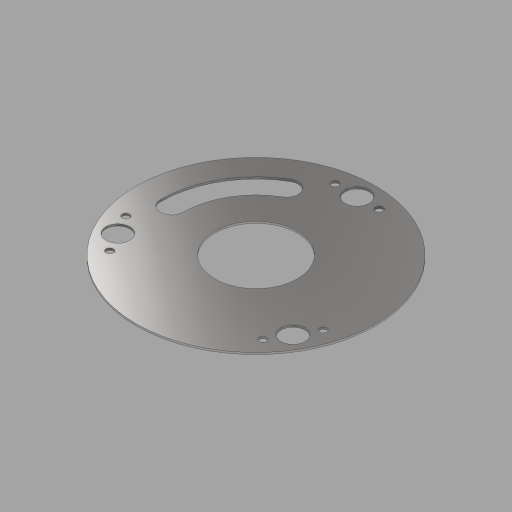
# Autodesk Inventor part: Baffle
Saved by Autodesk Inventor 2024 (Build 280153020, 153B)
## iProperties
Created: 2023-10-26
Part Number: Baffle
Material: Stainless Steel
Document SubType Name: Modeling
Designer: schanen
Density: 8 g/cm^3
Appearance: Semi-Polished
Mass: 11.1966 g
Surface Area: 231.347 cm^2
Volume: 11.1966 cm^3
baffle_or: 65.000 mm
tubes_r: 55.000 mm
Author: schanen
Autodesk Inventor part; units mm, degrees
ref_plane "YZ Plane" through (0, 0, 0) normal (1, 0, 0) x (0, 1, 0)
ref_plane "XZ Plane" through (0, 0, 0) normal (0, 1, 0) x (-1, 0, 0)
ref_plane "XY Plane" through (0, 0, 0) normal (0, 0, 1) x (1, 0, 0)
sketch "Sketch1" plane through (0, 0, 0) normal (0, 0, 1) x (1, 0, 0)
  line L0 (0, 0) -> (-65, 0)
  line L1 (-65, 0) -> (-65, 1)
  line L2 (-65, 1) -> (0, 1)
  line L3 (0, 1) -> (0, 0)
  dimension "baffle_or" = 65
  dimension "d1" = 1
  constraints: 8 end point, 2 parallel, 1 horizontal, 1 perpendicular
  measures "baffle_or" distance of L1.end L2.end
  measures "d1" distance of L0.end L1.end
revolve "Revolution1" add sketch "Sketch1" angle 360 about axis through (0, 1, 0) along (0, -1, 0)
sketch "Sketch2" plane through (0, 1, 0) normal (0, 1, 0) x (1, 0, 0)
  circle A0 centre (0, 0) radius 22.5
  dimension "d3" = 45
  constraints: 1 centre point, 1 coincident
  measures "d3" diameter of A0
extrude "Extrusion1" cut sketch "Sketch2" against normal through all
sketch "Sketch3" plane through (0, 1, 0) normal (0, 1, 0) x (1, 0, 0)
  circle A0 centre (0, 55) radius 6.5
  circle A1 centre (-12, 55) radius 2
  circle A2 centre (12, 55) radius 2
  point P0 (0, 0)
  dimension "d12" = 13
  dimension "tubes_r" = 55
  dimension "d14" = 4
  dimension "d15" = 12
  dimension "d16" = 4
  dimension "d17" = 12
  constraints: 3 centre point, 2 horizontal alignment, 1 vertical alignment
  measures "d12" diameter of A0
  measures "tubes_r" distance of point (0, 0) A0.centre
  measures "d14" diameter of A1
  measures "d15" distance of A1.centre A0.centre
  measures "d16" diameter of A2
  measures "d17" distance of A2.centre A0.centre
extrude "Extrusion2" cut sketch "Sketch3" against normal through all
pattern_circular "Circular Pattern1" count 3 over 360 about axis through (0, 1, 0) along (0, -1, 0) of "Extrusion2"
sketch "Sketch4" plane through (0, 1, 0) normal (0, 1, 0) x (1, 0, 0)
  arc A0 (-23, 39.8372) -> (-46, 0) centre (0, 0) ccw construction
  arc A1 (-26, 45.0333) -> (-52, 0) centre (0, 0) ccw
  arc A2 (-20, 34.641) -> (-40, 0) centre (0, 0) ccw
  arc A3 (-20, 34.641) -> (-26, 45.0333) centre (-23, 39.8372) ccw
  arc A4 (-52, 0) -> (-40, 0) centre (-46, 0) ccw
  line L0 (0, 0) -> (-23, 39.8372) construction
  line L1 (0, 0) -> (-46, 0) construction
  circle A5 centre (0, 55) radius 6.5 projected
  line L2 (0, 0) -> (0, 55) construction
  circle A6 centre (-47.6314, -27.5) radius 6.5 projected
  line L3 (0, 0) -> (-47.6314, -27.5) construction
  dimension "d23" = 60
  dimension "d24" = 30
  dimension "d25" = 30
  dimension "d26" = 6
  dimension "d27" = 40
  constraints: 10 point on circle, 8 end point, 5 centre point, 4 tangent, 1 coincident, 1 vertical
  measures "d23" angle of L1 L0
  measures "d24" angle of L0 L2
  measures "d25" angle of L3 L1
  measures "d26" radius of A4
  measures "d27" radius of A2
extrude "Extrusion3" cut sketch "Sketch4" against normal through all contours A3 A2 A4 A1
equation "\"d17\" = d15"
body "Solid1"
